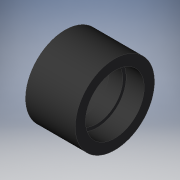
# Autodesk Inventor part: C-AFBD22-35W_bw
Saved by Autodesk Inventor 2019 (Build 230136000, 136)
## iProperties
Created: 2023-11-09
Part Number: C-AFBD22-35W_bw
Material: Generic
Catalog Web Link: www.cadenas.de
Description: C-AFBD-W, C-AFDF-W_bw-Economy Idlers Backside Tension Type
Vendor: MISUMI
Document SubType Name: Modeling
Designer: psAdmin
Manufacturer: MISUMI
Mass: 10.1788 g
Surface Area: 52.5274 cm^2
Volume: 10.1788 cm^3
Density: 1 g/cm^3
Appearance: PSOLRGB-175-175-175
Category: PARTsolutions
Company: MISUMI
Title: C-AFBD22-35W
Author: Cadenas PARTsolutions
Comments: Economy Idlers Backside Tension Type
PSOL_IDENT_0: {$CADENAS_DATA/23d-libs/misumi/metric/51_timing_pulleys/c_afbd/c_afbd_w_body.prj},185 {VTYP=3D},{NB=
PSOL_IDENT_1: C-AFBD22-35W_bw},{LINA=C-AFBD22-35W},{NN=C-AFBD-W, C-AFDF-W_bw},{DATE=13.09.2022 06:55:24},{GEOMDATE=
PSOL_IDENT_2: 18.05.2021 06:11:19},{VERSION=},{LINEID=100},{WBVAR=TS},{WBNUMERIC=}  {NB=C-AFBD22-35W_bw},{LINA=C-A
PSOL_IDENT_3: FBD22-35W},{KT=DUMMY},{PN=C-AFBD22-35W},{TYPE=C-AFBD},{TS=C-AFBD},{TSALG= 'C-AFBD','No Flange','C-AF
PSOL_IDENT_4: DF','Flanged' },{W=22},{NOM=35W},{NOMALG= '25','35W' },{D=35},{F=45},{A=17},{ABI=-},{ABM=150},{NO=60
PSOL_IDENT_5: 00ZZ×2},{BN=6000},{DD=10},{B=8.0},{E=30.000},{BD=26.000},{DH=23.000},{PTT=1.000},{CIF=2.000}
NB: C-AFBD22-35W_bw
NN: C-AFBD-W, C-AFDF-W_bw
NT: Economy Idlers Backside Tension Type
NBSYN: $PN._bw
LINA: C-AFBD22-35W
CATALOG: Misumi
PN: C-AFBD22-35W
TYPE: C-AFBD
TS: No Flange
W: 22
NOM: 35W
D: 35
F: 45
A: 17
ABI: -
ABM: 150
NO: 6000ZZ×2
BN: 6000
DD: 10
B: 8
SUPPLIER: MISUMI
ARTICLENO: C-AFBD22-35W_bw
BOMINFO: C-AFBD22-35W
CREATOR: CADENAS GmbH
Autodesk Inventor part; units mm, degrees
sketch "_____1" plane through (0, 0, 0) normal (0, 0, 1) x (1, 0, 0)
  line L0 (11, 0) -> (-11, 0)
  line L1 (-11, 0) -> (-11, 17.5)
  line L2 (-11, 17.5) -> (11, 17.5)
  line L3 (11, 17.5) -> (11, 0)
  line L4 (11, 0) -> (-11, 0)
  constraints: 10 end point
revolve "Revolution1" add sketch "_____1" angle 360 about axis through (11, 0, 0) along (1, 0, 0)
sketch "_____3" plane through (0, 0, 0) normal (0, 0, 1) x (1, 0, 0)
  line L0 (11, 0) -> (-11, 0)
  line L1 (-11, 0) -> (-11, 13)
  line L2 (-11, 13) -> (-3, 13)
  line L3 (-3, 13) -> (-3, 11.5)
  line L4 (-3, 11.5) -> (3, 11.5)
  line L5 (3, 11.5) -> (3, 13)
  line L6 (3, 13) -> (11, 13)
  line L7 (11, 13) -> (11, 0)
  line L8 (11, 0) -> (-11, 0)
  constraints: 18 end point
revolve "Revolution2" cut sketch "_____3" angle 360 about axis through (11, 0, 0) along (1, 0, 0)
ref_plane "b6000_1_XY" through (7, 0, 0) normal (1, 0, 0) x (0, 0, -1)
ref_plane "b6000_1_YZ" through (7, 0, 0) normal (0, 0, -1) x (0, 1, 0)
ref_plane "b6000_1_ZX" through (7, 0, 0) normal (0, 1, 0) x (1, 0, 0)
ref_plane "b6000_2_XY" through (-7, 0, 0) normal (1, 0, 0) x (0, 0, -1)
ref_plane "b6000_2_YZ" through (-7, 0, 0) normal (0, 0, -1) x (0, 1, 0)
ref_plane "b6000_2_ZX" through (-7, 0, 0) normal (0, 1, 0) x (1, 0, 0)
ref_plane "to_dummy_XY" through (0, 0, 0) normal (1, 0, 0) x (0, 0, -1)
ref_plane "to_dummy_YZ" through (0, 0, 0) normal (0, 0, -1) x (0, 1, 0)
ref_plane "to_dummy_ZX" through (0, 0, 0) normal (0, 1, 0) x (1, 0, 0)
body "Solid1"
